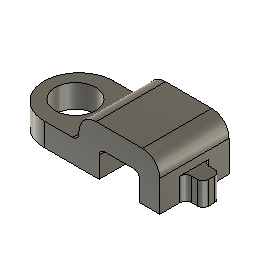
logger_mounting_reed_switch (Autodesk Fusion 360 design; units mm, degrees)
Autodesk Fusion 360 part; units mm, degrees
note: some values were not read from the file. Set by a fixed rule: which sketch regions a step uses; the direction of a hole.
sketch "Skizze8" plane through (0, 0, 0) normal (0, 1, 0) x (1, 0, 0)
  line L0 (-9.5, 0) -> (-1.75, 0)
  line L1 (-1.75, 0) -> (-1.75, -2.3)
  line L2 (-1.75, -2.3) -> (1.75, -2.3)
  line L3 (1.75, -2.3) -> (1.75, 0)
  line L4 (1.75, 0) -> (3.5, 0)
  line L5 (3.5, -2) -> (3.5, -4.2)
  line L6 (3.5, -4.2) -> (-3.5, -4.2)
  line L7 (-3.5, -4.2) -> (-3.5, -2)
  line L8 (-3.5, -2) -> (-9.5, -2)
  line L9 (-9.5, -2) -> (-9.5, 0)
  line L10 (3.5, 0) -> (5, 0)
  line L11 (5, 0) -> (5, -2)
  line L12 (5, -2) -> (3.5, -2)
  dimension "d100" = 3.5
  dimension "d101" = 1.75
  dimension "d102" = 2.3
  dimension "d103" = 7
  dimension "d104" = 3.5
  dimension "d105" = 4.2
  dimension "d110" = 2
  dimension "d123" = 6
  dimension "d134" = 1.5
  constraint perpendicular L0 L1
  constraint perpendicular L1 L2
  constraint perpendicular L2 L3
  constraint perpendicular L3 L4
  constraint perpendicular L5 L6
  constraint perpendicular L7 L8
  constraint perpendicular L0 L9
  constraint horizontal L0
  constraint horizontal origin L0.start
  constraint collinear L0 L4
  constraint perpendicular L6 L7
  constraint perpendicular L4 L11
  constraint equal L9 L11
  constraint perpendicular L5 L12
  constraint perpendicular L10 L11
  measures "d100" distance of L1 L3
  measures "d101" distance of origin L1
  measures "d102" distance of origin L2
  measures "d103" distance of L5.end L6.end
  measures "d104" distance of origin L5
  measures "d105" distance of origin L6
  measures "d110" distance of L0 L8
  measures "d123" distance of L7 L9
  measures "d134" distance of L5.start L11.end
extrude "Extrusion5" add sketch "Skizze8" along normal blind 6
sketch "Skizze9" plane through (0, 0, 0) normal (0, 0, 1) x (1, 0, 0)
  line L0 (-9.5, 0) -> (-9.5, 6)
  line L1 (-3.5, 0) -> (-9.5, 0)
  line L2 (-3.5, 0) -> (-3.5, 6)
  line L3 (0, 1.75) -> (0, 22.5)
  point P0 (-6.8, 3)
  point P1 (6.8, 3)
  dimension "d113" = 6
  dimension "d114" = 3
  dimension "d120" = 9.5
  dimension "d128" = 3.3
  constraint horizontal P0 P1
  constraint symmetric P0 P1 L3
  measures "d113" distance of L0.start L0.end
  measures "d114" distance of P0 L1
  measures "d120" distance of origin L0
  measures "d128" distance of P0 L2
hole "Bohrung4" at (-6.8, 3, 0) at (6.8, 3, 0) direction (0, 0, 1) diameter 3.5 depth 5 tip angle 118
fillet "Abrundung7" radius 3 2 edges at (-9.5, 0, 1) (-9.5, 6, 1)
fillet "Abrundung8" radius 0.55 1 edges at (-3.5, 3, 2)
fillet "Abrundung9" radius 0.5 2 edges at (-1.75, 3, 2.3) (1.75, 3, 2.3)
fillet "Abrundung10" radius 1.5 2 edges at (-3.5, 3, 4.2) (3.5, 3, 4.2)
sketch "Skizze10" plane through (0, 0, 0) normal (0, 0, 1) x (1, 0, 0)
  line L0 (3.5, 0) -> (5, 0)
  line L1 (5, 0) -> (5, 2.25)
  line L2 (5, 2.25) -> (3.5, 2.25)
  line L3 (3.5, 2.25) -> (3.5, 0)
  line L4 (3.5, 6) -> (5, 6)
  line L5 (5, 6) -> (5, 3.75)
  line L6 (5, 3.75) -> (3.5, 3.75)
  line L7 (3.5, 3.75) -> (3.5, 6)
  line L8 (3.5, 0) -> (5, 0)
  line L9 (5, 0) -> (5, 6)
  line L10 (5, 6) -> (3.5, 6)
  line L11 (3.5, 6) -> (3.5, 0)
  line L12 (3.5, 6) -> (5, 6)
  line L13 (5, 0) -> (3.5, 0)
  dimension "d135" = 1.5
  dimension "d136" = 1.5
  dimension "d141" = 1.5
  constraint horizontal L0
  constraint vertical L1
  constraint horizontal L2
  constraint vertical L3
  constraint horizontal L4
  constraint vertical L5
  constraint horizontal L6
  constraint vertical L7
  constraint coincident L5.end L9
  constraint coincident L4.start L10
  constraint coincident L0.start L13
  constraint coincident L1.end L9
  constraint equal L1 L5
  measures "d135" distance of L5.end L6.end
  measures "d136" distance of L1.end L2.end
  measures "d141" distance of L2 L6
extrude "Extrusion6" cut sketch "Skizze10" along normal up to surface (2 mm away) contours L0 L1 L2 L3 L8 L9 L11 L13 | L4 L5 L6 L7 L9 L10 L11 L12
fillet "Abrundung11" radius 0.5 4 edges at (3.5, 2.25, 1) (3.5, 3.75, 1) (5, 2.25, 1) (5, 3.75, 1)
equation "d101 = d100 / 2"
equation "d104 = d103 / 2"
equation "d106 = 2 mm"
equation "d110 = d106"
equation "d114 = d113 / 2"
